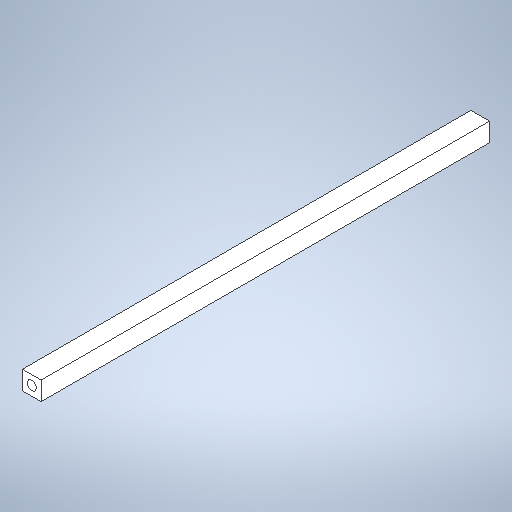
# Autodesk Inventor part: 回収機構スペーサ
Saved by Autodesk Inventor 2026.2 (Build 302298010, 298A)
## iProperties
Created: 2026-05-06
Part Number: 回収機構スペーサ
Material: 一般
Document SubType Name: Modeling
Designer: Yagis
Density: 1 g/cm^3
Appearance: 既定
Author: Yagis
Autodesk Inventor part; units mm, degrees
ref_plane "YZ Plane" through (0, 0, 0) normal (1, 0, 0) x (0, 1, 0)
ref_plane "XZ Plane" through (0, 0, 0) normal (0, 1, 0) x (-1, 0, 0)
ref_plane "XY Plane" through (0, 0, 0) normal (0, 0, 1) x (1, 0, 0)
sketch "スケッチ1" plane through (0, 0, 0) normal (0, 0, 1) x (1, 0, 0)
  line L0 (-2.5, 2.5) -> (2.5, 2.5)
  line L1 (2.5, 2.5) -> (2.5, -2.5)
  line L2 (2.5, -2.5) -> (-2.5, -2.5)
  line L3 (-2.5, -2.5) -> (-2.5, 2.5)
  point P0 (0, 0)
  point P1 (-2.5, 0)
  point P2 (0, 2.5)
  dimension "d4" = 5
  dimension "d5" = 5
  constraints: 8 end point, 2 midpoint, 2 parallel, 1 horizontal, 1 horizontal alignment, 1 perpendicular, 1 vertical alignment
  measures "d4" distance of L0.start L0.end
  measures "d5" distance of L0.end L1.end
extrude "押し出し1" add sketch "スケッチ1" along normal blind 120
sketch "スケッチ2" plane through (0, 0, 120) normal (0, 0, 1) x (1, 0, 0)
  point P0 (0, 0)
hole "穴1" at (0, 0, 120) direction (0, 0, -1) diameter 2.459 depth 8.8 tip angle 118 thread size "M3x0.5" class "6H" standard "ISO Metric profile"
sketch "スケッチ3" plane through (0, 0, 0) normal (0, 0, -1) x (-1, 0, 0)
  point P0 (0, 0)
  point P1 (0, 0)
  constraints: 1 coincident
hole "穴2" at (0, 0, 0) direction (0, 0, 1) diameter 2.459 depth 8.8 tip angle 118 thread size "M3x0.5" class "6H" standard "ISO Metric profile"
